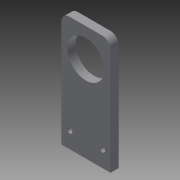
# Autodesk Inventor part: arm mount
Saved by Autodesk Inventor 2013 (Build 170138000, 138)
## iProperties
Created: 2013-01-20
Part Number: arm mount
Material: Generic
Document SubType Name: Sheet Metal
Designer: Arpan
Density: 1 g/cm^3
Sheet Metal Rule: Default
Author: Arpan
Autodesk Inventor part; units mm, degrees
ref_plane "YZ Plane" through (0, 0, 0) normal (1, 0, 0) x (0, 1, 0)
ref_plane "XZ Plane" through (0, 0, 0) normal (0, 1, 0) x (-1, 0, 0)
ref_plane "XY Plane" through (0, 0, 0) normal (0, 0, 1) x (1, 0, 0)
sketch "Sketch1" plane through (0, 0, 0) normal (0, 0, 1) x (1, 0, 0)
  line L0 (0, 0) -> (-38.1, 0)
  line L1 (0, 0) -> (0, 82.55)
  line L2 (-6.35, 88.9) -> (-38.1, 88.9)
  line L3 (-38.1, 82.55) -> (-38.1, 0)
  line L4 (-31.75, 88.9) -> (-31.75, 88.9)
  line L5 (-31.75, 88.9) -> (-31.75, 12.7)
  line L6 (0, 88.9) -> (-6.35, 88.9)
  line L7 (-6.35, 88.9) -> (-6.35, 12.7)
  circle A0 centre (-31.75, 12.7) radius 2.1463
  circle A1 centre (-6.35, 12.7) radius 2.1463
  arc A2 (-31.75, 88.9) -> (-38.1, 82.55) centre (-31.75, 82.55) ccw
  arc A3 (0, 82.55) -> (-6.35, 88.9) centre (-6.35, 82.55) ccw
  line L8 (-22.225, 88.9) -> (-22.225, 63.5)
  dimension "d0" = 38.1
  dimension "d1" = 88.9
  dimension "d2" = 6.35
  dimension "d3" = 76.2
  dimension "d4" = 6.35
  dimension "d5" = 4.2926
  dimension "d6" = 4.2926
  dimension "d7" = 76.2
  dimension "d19" = 6.35
  dimension "d20" = 6.35
  dimension "d23" = 25.4
  measures "d0" distance of L0.start L0.end
  measures "d1" distance of L0.start L6.start
  measures "d2" distance of L2.end L4.end
  measures "d3" distance of L4.end L5.end
  measures "d4" distance of L6.start L6.end
  measures "d5" diameter of A0
  measures "d6" diameter of A1
  measures "d7" distance of L6.end L7.end
  measures "d19" radius of A2
  measures "d20" radius of A3
  measures "d23" distance of L8.start L8.end
extrude "Plate1" add sketch "Sketch1" along normal blind 6.35
sketch "Sketch4" plane through (0, 0, 0) normal (0, 0, -1) x (-1, 0, 0)
  line L0 (6.35, 88.9) -> (31.75, 88.9) projected
  line L1 (19.05, 88.9) -> (19.05, 66.675)
  circle A0 centre (19.05, 66.675) radius 14.2875
  dimension "d25" = 22.225
  dimension "d26" = 28.575
  constraints: 2 end point, 1 centre point, 1 coincident, 1 midpoint, 1 perpendicular
  measures "d25" distance of L1.start L1.end
  measures "d26" diameter of A0
extrude "Cut1" cut sketch "Sketch4" against normal blind 6.35
equation "\"d27\" = Thickness"
equation "\"BendRadius\" = Thickness"
equation "\"BendReliefWidth\" = Thickness"
equation "\"BendReliefDepth\" = 0.5 * Thickness"
equation "\"CornerReliefSize\" = 4 * Thickness"
equation "\"MinimumRemnant\" = 2 * Thickness"
equation "\"TransitionRadius\" = BendRadius"
equation "\"JacobiRadiusSize\" = BendRadius"
equation "\"GapSize\" = Thickness"
equation "\"d8\" = BendRadius"
equation "\"Thickness\" = 6.35"
body "Solid1"
